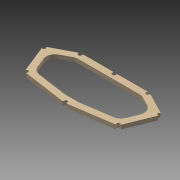
# Autodesk Inventor part: section1
Saved by Autodesk Inventor 2015 (Build 190159000, 159)
## iProperties
Created: 2017-09-23
Part Number: section1
Material: Polyethylene, High Density
Document SubType Name: Modeling
Designer: Mimoja
Density: 0.952 g/cm^3
Appearance: Smooth - Off-White
Mass: 553.113 g
Surface Area: 1075.49 cm^2
Volume: 581.001 cm^3
Author: Mimoja
Autodesk Inventor part; units mm, degrees
ref_plane "YZ Plane" through (0, 0, 0) normal (1, 0, 0) x (0, 1, 0)
ref_plane "XZ Plane" through (0, 0, 0) normal (0, 1, 0) x (-1, 0, 0)
ref_plane "XY Plane" through (0, 0, 0) normal (0, 0, 1) x (1, 0, 0)
sketch "Sketch1" plane through (0, 0, 0) normal (0, 0, 1) x (1, 0, 0)
  line L0 (0, 2.1336) -> (-207.5688, 32.6136)
  line L1 (-207.5688, 32.6136) -> (-263.0424, 170.9928)
  line L2 (-263.0424, 170.9928) -> (-152.4, 228.6)
  line L3 (0, 569.8709) -> (0, -138.2601) construction
  line L4 (-152.4, 228.6) -> (0, 228.6)
  line L5 (0, 228.6) -> (0, 2.1336)
  point P0 (0, 0)
  dimension "d9" = 228.6
  dimension "d11" = 263.0424
  dimension "d15" = 170.9928
  dimension "d20" = 207.5688
  dimension "d22" = 32.6136
  dimension "d39" = 152.4
  dimension "d41" = 0
  dimension "d42" = 2.1336
  constraints: 12 end point, 1 collinear, 1 perpendicular, 1 point on line, 1 vertical
  measures "d9" vertical distance of point (0, 0) L2.end
  measures "d11" horizontal distance of point (0, 0) L1.end
  measures "d15" vertical distance of point (0, 0) L1.end
  measures "d20" horizontal distance of point (0, 0) L0.end
  measures "d22" vertical distance of point (0, 0) L0.end
  measures "d39" horizontal distance of point (0, 0) L2.end
  measures "d41" horizontal distance of point (0, 0) L0.start
  measures "d42" distance of point (0, 0) L0.start
extrude "Extrusion4" add sketch "Sketch1" along normal blind 18
hole "Hole2" at (0.0182, 221.5256, 18) direction (0, 0, -1) diameter 15 end through all
hole "Hole3" at (-256.2008, 168.2751, 18) direction (0, 0, -1) diameter 15 end through all
hole "Hole4" at (-203.4994, 38.3667, 18) direction (0, 0, -1) diameter 15 end through all
hole "Hole5" at (0.2097, 9.0005, 18) direction (0, 0, -1) diameter 15 end through all
hole "Hole6" at (-150.3581, 221.9476, 18) direction (0, 0, -1) diameter 15 end through all
fillet "Fillet6" radius 5 1 edges at (-2.4724, 228.6, 9)
fillet "Fillet7" radius 3 1 edges at (-146.8946, 228.6, 9)
fillet "Fillet8" radius 3 1 edges at (-156.2403, 226.6005, 9)
fillet "Fillet9" radius 1 1 edges at (-254.3184, 175.535, 9)
fillet "Fillet10" radius 1 1 edges at (-259.1966, 161.3994, 9)
fillet "Fillet11" radius 3.5 1 edges at (-3.8594, 2.7003, 9)
fillet "Fillet12" radius 1 1 edges at (-210.7068, 40.4413, 9)
fillet "Fillet13" radius 1 1 edges at (-200.3605, 31.5551, 9)
sketch "Sketch4" plane through (0, 0, 18) normal (0, 0, 1) x (1, 0, 0)
  line L0 (-30, 34.8392) -> (-187.5705, 57.9773)
  line L1 (-187.5705, 57.9773) -> (-227.6157, 157.8702)
  line L2 (-227.6157, 157.8702) -> (-145.5473, 200.6)
  line L3 (-145.5473, 200.6) -> (0, 200.6)
  line L4 (0, 16.4976) -> (0, 214.0256) projected
  line L5 (-30, 34.8392) -> (0, 34.8392)
  line L6 (0, 200.6) -> (0, 34.8392)
  line L7 (-162.1854, 223.5051) -> (-252.4163, 176.5254) projected
  line L8 (-12.3085, 228.6) -> (-140.5138, 228.6) projected
  line L9 (-258.4369, 159.5042) -> (-211.572, 42.5997) projected
  line L10 (-197.8243, 31.1827) -> (-11.1561, 3.7718) projected
  point P0 (0, 0)
  dimension "d175" = 28
  dimension "d176" = 28
  dimension "d177" = 28
  dimension "d178" = 28
  dimension "d179" = 30
  constraints: 12 end point, 4 parallel, 2 horizontal, 2 point on line, 1 collinear
  measures "d175" distance between parallel lines of L2 L7
  measures "d176" distance between parallel lines of L8 L3
  measures "d177" distance between parallel lines of L1 L9
  measures "d178" distance between parallel lines of L10 L0
  measures "d179" distance of L0.start L5.end
extrude "Extrusion5" cut sketch "Sketch4" against normal through all
fillet "Fillet14" radius 40 1 edges at (-227.6157, 157.8702, 9)
fillet "Fillet15" radius 40 1 edges at (-187.5705, 57.9773, 9)
fillet "Fillet16" radius 40 1 edges at (-145.5473, 200.6, 9)
fillet "Fillet17" radius 40 1 edges at (-30, 34.8392, 9)
mirror "Mirror3" about plane through (0, 0, 0) normal (1, 0, 0)
body "Solid4"
